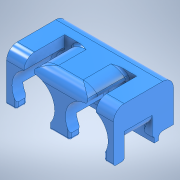
# Autodesk Inventor part: Belt_Clamp
Saved by Autodesk Inventor 2021 (Build 250183000, 183)
## iProperties
Created: 2021-11-16
Part Number: Belt_Clamp
Material: Generic
Document SubType Name: Modeling
Designer: Jorian Brusind
Density: 1 g/cm^3
Appearance: Cyan
Author: Jorian Brusind
Autodesk Inventor part; units mm, degrees
ref_plane "YZ Plane" through (0, 0, 0) normal (1, 0, 0) x (0, 1, 0)
ref_plane "XZ Plane" through (0, 0, 0) normal (0, 1, 0) x (-1, 0, 0)
ref_plane "XY Plane" through (0, 0, 0) normal (0, 0, 1) x (1, 0, 0)
sketch "Sketch1" plane through (0, 0, 0) normal (0, 1, 0) x (-1, 0, 0)
  line L0 (0, 0) -> (50, 0)
  line L1 (50, 0) -> (50, -28)
  line L2 (50, -28) -> (0, -28)
  line L3 (0, -28) -> (0, 0)
  dimension "d0" = 50
  dimension "d1" = 28
  constraints: 8 end point, 2 parallel, 1 horizontal, 1 perpendicular
  measures "d0" distance of L1.end L2.end
  measures "d1" distance of L0.end L1.end
extrude "Extrusion1" add sketch "Sketch1" along normal blind 20
sketch "Sketch2" plane through (-50, 0, 0) normal (0, 0, 1) x (1, 0, 0)
  line L0 (50, 0) -> (0, 0) projected
  line L1 (25, 0) -> (12.5, 0)
  line L2 (12.5, 0) -> (12.5, 6)
  line L3 (50, 20) -> (0, 20) projected
  circle A0 centre (12.5, 6) radius 10
  line L4 (25, 0) -> (37.5, 0)
  line L5 (37.5, 0) -> (37.5, 6)
  circle A1 centre (37.5, 6) radius 10
  circle A2 centre (12.5, 6) radius 3
  circle A3 centre (37.5, 6) radius 3
  point P0 (20.5, 0)
  point P1 (4.5, 0)
  point P2 (45.5, 0)
  point P3 (29.5, 0)
  dimension "d4" = 12.5
  dimension "d5" = 6
  dimension "d6" = 20
  dimension "d7" = 12.5
  dimension "d8" = 6
  dimension "d9" = 20
  dimension "d10" = 6
  dimension "d11" = 6
  constraints: 8 end point, 4 centre point, 4 coincident, 2 perpendicular, 2 point on line, 1 midpoint
  measures "d4" distance of L1.start L1.end
  measures "d5" distance of L1.end L2.end
  measures "d6" diameter of A0
  measures "d7" distance of L1.start L4.end
  measures "d8" distance of L4.end L5.end
  measures "d9" diameter of A1
  measures "d10" diameter of A2
  measures "d11" diameter of A3
extrude "Extrusion2" cut sketch "Sketch2" against normal blind 19 contours L0 A1 | L0 A0 | A2 | A3 picked at (40.7902, 1.2182) picked at (15.7902, 1.2182)
sketch "Sketch3" plane through (-50, 0, -19) normal (0, 0, 1) x (1, 0, 0)
  arc A0 (20.5, 0) -> (4.5, 0) centre (12.5, 6) ccw projected
  circle A1 centre (12.5, 6) radius 3.5
  arc A2 (45.5, 0) -> (29.5, 0) centre (37.5, 6) ccw projected
  circle A3 centre (37.5, 6) radius 3.5
  point P0 (50, 0)
  dimension "d14" = 7
  dimension "d15" = 7
  constraints: 2 centre point, 2 coincident
  measures "d14" diameter of A1
  measures "d15" diameter of A3
extrude "Extrusion3" cut sketch "Sketch3" against normal through all
sketch "Sketch4" plane through (0, 0, 0) normal (0, -1, 0) x (1, 0, 0)
  line L0 (-50, -28) -> (-50, 0) projected
  line L1 (-50, -28) -> (0, -28)
  line L2 (0, -28) -> (0, 0)
  line L3 (0, 0) -> (-50, 0)
  line L4 (-50, 0) -> (-50, -28)
  line L5 (0, 0) -> (0, -28) projected
  line L6 (-50, 0) -> (0, 0)
  line L7 (0, 0) -> (0, -21)
  line L8 (0, -21) -> (-50, -21)
  line L9 (-50, -21) -> (-50, 0)
  line L10 (-48, -19) -> (-2, -19)
  line L11 (-2, -19) -> (-2, -2)
  line L12 (-2, -2) -> (-48, -2)
  line L13 (-48, -2) -> (-48, -19)
  line L14 (-48, -19) -> (-50, -19)
  line L15 (-48, -2) -> (-50, -2)
  line L16 (-2, -19) -> (0, -19)
  line L17 (-2, -2) -> (0, -2)
  line L18 (-45.5, -19) -> (-45.5, 0) projected
  line L19 (-45.5, -19) -> (-45.5, -2)
  line L20 (-45.5, -2) -> (-45.5, 0)
  line L21 (-29.5, 0) -> (-29.5, -19) projected
  line L22 (-29.5, 0) -> (-20.5, 0) projected
  line L23 (-29.5, -19) -> (-29.5, 0)
  line L24 (-29.5, 0) -> (-29.5, -2)
  line L25 (-20.5, -19) -> (-20.5, 0) projected
  line L26 (-20.5, -19) -> (-20.5, 0)
  line L27 (-20.5, 0) -> (-20.5, -2)
  line L28 (-4.5, 0) -> (-4.5, -19) projected
  line L29 (-4.5, -19) -> (-4.5, 0)
  line L30 (-4.5, 0) -> (-4.5, -2)
  line L31 (-50, 0) -> (0, 0) projected
  line L32 (0, 0) -> (-50, 0)
  line L33 (-50, 0) -> (-50, -5)
  line L34 (-50, -5) -> (0, -5)
  line L35 (0, -5) -> (0, 0)
  line L36 (-45.5, -5) -> (-45.5, -2)
  line L37 (-29.5, -5) -> (-29.5, -2)
  line L38 (-20.5, -5) -> (-20.5, -2)
  line L39 (-4.5, -5) -> (-4.5, -2)
  line L40 (0, -5) -> (0, -2)
  point P0 (0, -19)
  point P1 (0, -21)
  point P2 (-4.5, -2)
  point P3 (-20.5, -2)
  point P4 (-29.5, -2)
  point P5 (-20.5, -5)
  point P6 (-45.5, -5)
  dimension "d18" = 21
  dimension "d19" = 2
  dimension "d38" = 5
  constraints: 66 end point, 26 point on line, 10 parallel, 7 perpendicular, 4 horizontal, 3 collinear, 1 vertical, 4 other
  measures "d18" distance of L6.end L7.end
  measures "d19" distance between parallel lines of L8 L10
  measures "d38" distance of L33.end L32.end
extrude "Extrusion4" add sketch "Sketch4" along normal blind 3 contours L0 L14 L10 L16 L2 L8 | L0 L15 L13 L34 | L0 L3 L18 L12 L15 | L13 L12 L18 L34 | L34 L11 L17 L2 | L17 L12 L28 L3 L2 | L34 L28 L12 L11 | L21 L12 L25 L34 | L3 L25 L12 L21
fillet "Fillet1" radius 1 4 edges at (-4.5, 0, -12) (-20.5, 0, -12) (-45.5, 0, -12) (-29.5, 0, -12)
fillet "Fillet4" radius 2 1 edges at (-25, 0, -21)
fillet "Fillet5" radius 1 3 edges at (-45.5, -3, -2.5) (-20.5, -3, -2.5) (-4.5, -3, -2.5)
fillet "Fillet6" radius 5 2 edges at (-25, 20, -28) (-25, 20, 0)
fillet "Fillet7" radius 1 2 edges at (-16, 6, -28) (-41, 6, -28)
fillet "Fillet8" radius 1 2 edges at (-41, 6, -19) (-16, 6, -19)
sketch "Sketch5" plane through (-29.3586, -3, 0) normal (0, 0, 1) x (1, 0, 0)
  line L0 (29.3586, 18) -> (-20.6414, 18) projected
  line L1 (-20.6414, 18) -> (-12.5003, 18)
  arc A0 (0.24, 3.5455) -> (-16.5228, 3.5455) centre (-8.1414, 9) ccw projected
  line L2 (-20.6414, 23) -> (29.3586, 23) projected
  line L3 (-12.5003, 18) -> (-9.5003, 18)
  line L4 (-9.5003, 18) -> (-9.5003, 23)
  line L5 (-9.5003, 23) -> (-12.5003, 23)
  line L6 (-12.5003, 23) -> (-12.5003, 18)
  line L7 (29.3586, 0) -> (-20.6414, 0) projected
  line L8 (4.3586, 0) -> (4.3586, 23)
  line L9 (21.2175, 18) -> (18.2175, 18)
  line L10 (18.2175, 18) -> (18.2175, 23)
  line L11 (18.2175, 23) -> (21.2175, 23)
  line L12 (21.2175, 23) -> (21.2175, 18)
  point P0 (29.3586, 3)
  point P1 (21.2175, 18)
  point P2 (21.2175, 23)
  point P3 (18.2175, 23)
  point P4 (18.2175, 18)
  point P5 (-9.5003, 18.9072)
  dimension "d30" = 3
  constraints: 20 end point, 4 symmetric about line, 2 horizontal, 2 midpoint, 2 parallel, 1 perpendicular, 1 point on circle, 1 point on line
  measures "d30" distance of L5.end L4.end
extrude "Extrusion5" cut sketch "Sketch5" against normal up to surface (19 mm away) contours L0 L10 L2 L12 | A0 L6 L2 L4
fillet "Fillet9" radius 10 4 edges at (-38.8589, 18.8429, -1.8013) (-38.8589, 20, -12) (-11.1411, 18.8429, -1.8013) (-11.1411, 20, -12)
fillet "Fillet10" radius 1 2 edges at (-11.1411, 15.9072, -9.5415) (-38.8589, 15.9072, -9.5415)
fillet "Fillet11" radius 1 9 edges at (-28.5548, 0.4778, -19) (-25, 0, -19) (-21.4452, 0.4778, -19) (-21.2562, 10.8299, -19) (-12.5416, 16.6607, -19) (-15.839, 19.4147, -19) (-37.4584, 16.6607, -19) (-34.161, 19.4147, -19) (-28.7438, 10.8299, -19)
fillet "Fillet12" radius 1 3 edges at (-3.5548, 0.4778, -19) (-1.351, 0, -19) (-3.0202, 9.1832, -19)
fillet "Fillet13" radius 1 3 edges at (-46.4452, 0.4778, -19) (-48.649, 0, -19) (-46.9798, 9.1832, -19)
fillet "Fillet14" radius 1 18 edges at (-45.7929, -2.7071, -5) (-45.5, -1, -5) (-48.25, -3, -5) (-45.7929, -2.7071, 0) (-45.5, -1, 0) (-48.25, -3, 0) (-20.7929, -2.7071, -5) (-20.5, -1, -5) (-25.5, -3, -5) (-20.7929, -2.7071, 0) (-20.5, -1, 0) (-25.5, -3, 0) (-4.2071, -2.7071, -5) (-4.5, -1, -5) (-1.75, -3, -5) (-4.2071, -2.7071, 0) (-4.5, -1, 0) (-1.75, -3, 0)
sketch "Sketch6" plane through (-50, -3, -21) normal (-1, 0, 0) x (0, 0, 1)
  line L0 (3, 3) -> (16, 3) projected
  line L1 (16, 3) -> (3, 3)
  line L2 (3, 3) -> (3, 8)
  line L3 (3, 8) -> (16, 8)
  line L4 (16, 8) -> (16, 3)
  point P0 (21, 3)
  point P1 (3, 3)
  dimension "d40" = 13
  dimension "d41" = 5
  constraints: 8 end point, 2 parallel, 1 horizontal, 1 perpendicular
  measures "d40" distance of L2.end L3.end
  measures "d41" distance of L1.end L2.end
extrude "Extrusion6" cut sketch "Sketch6" against normal through all
fillet "Fillet15" radius 4 2 edges at (-50, 5, -11.5) (0, 5, -11.5)
body "Solid1"
